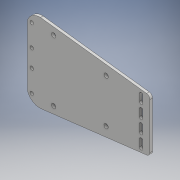
# Autodesk Inventor part: SoporteMano
Saved by Autodesk Inventor 2018 (Build 220112000, 112)
## iProperties
Created: 2017-10-02
Part Number: SoporteMano
Material: Genérico
Document SubType Name: Modeling
Designer: Pablo
Density: 1 g/cm^3
Appearance: Valor por defecto
Author: Pablo
Autodesk Inventor part; units mm, degrees
ref_plane "YZ Plane" through (0, 0, 0) normal (1, 0, 0) x (0, 1, 0)
ref_plane "XZ Plane" through (0, 0, 0) normal (0, 1, 0) x (-1, 0, 0)
ref_plane "XY Plane" through (0, 0, 0) normal (0, 0, 1) x (1, 0, 0)
sketch "Boceto1" plane through (0, 0, 0) normal (0, 1, 0) x (-1, 0, 0)
  line L0 (125, 0) -> (125, 45)
  line L1 (140, 0) -> (140, 35)
  arc A0 (140, 35) -> (125, 45) centre (125.919, 30.1285) ccw
  line L2 (0, 0) -> (0, 26.2041)
  line L3 (10, 0) -> (10, 32.2222)
  line L4 (0, 0) -> (0, 7.5)
  line L5 (0, 7.5) -> (0, 22.5)
  arc A1 (8, 3.5) -> (12, 3.5) centre (10, 3.5) ccw
  line L6 (10, 7.5) -> (6.5727, 7.5)
  arc A2 (12, 11.5) -> (8, 11.5) centre (10, 11.5) ccw
  line L7 (10, 15) -> (5.5099, 15)
  line L8 (12, 11.5) -> (12, 3.5)
  line L9 (8, 3.5) -> (8, 11.5)
  arc A3 (12, 26.5) -> (8, 26.5) centre (10, 26.5) ccw
  arc A4 (8, 18.5) -> (12, 18.5) centre (10, 18.5) ccw
  line L10 (12, 18.5) -> (12, 26.5)
  line L11 (8, 26.5) -> (8, 18.5)
  circle A5 centre (135, 10) radius 2
  circle A6 centre (135, 35) radius 2
  circle A7 centre (110, 35) radius 2.5
  line L12 (125, 45) -> (3.7689, 30.4523)
  circle A8 centre (50, 25) radius 2.5
  arc A9 (3.7689, 30.4523) -> (0, 26.2041) centre (4.2786, 26.2041) ccw
  line L13 (0, 0) -> (10, 0)
  line L14 (125, 0) -> (125, -45)
  line L15 (140, 0) -> (140, -35)
  arc A10 (125, -45) -> (140, -35) centre (125.919, -30.1285) ccw
  line L16 (0, 0) -> (0, -26.2041)
  line L17 (10, 0) -> (10, -32.2222)
  line L18 (0, 0) -> (0, -7.5)
  line L19 (0, -7.5) -> (0, -22.5)
  arc A11 (12, -3.5) -> (8, -3.5) centre (10, -3.5) ccw
  line L20 (10, -7.5) -> (6.5727, -7.5)
  arc A12 (8, -11.5) -> (12, -11.5) centre (10, -11.5) ccw
  line L21 (10, -15) -> (5.5099, -15)
  line L22 (12, -11.5) -> (12, -3.5)
  line L23 (8, -3.5) -> (8, -11.5)
  arc A13 (12, -18.5) -> (8, -18.5) centre (10, -18.5) ccw
  line L24 (12, -18.5) -> (12, -26.5)
  line L25 (8, -26.5) -> (8, -18.5)
  arc A14 (8, -26.5) -> (12, -26.5) centre (10, -26.5) ccw
  circle A15 centre (135, -10) radius 2
  circle A16 centre (135, -35) radius 2
  circle A17 centre (110, -35) radius 2.5
  line L26 (125, -45) -> (3.7689, -30.4523)
  circle A18 centre (50, -25) radius 2.5
  arc A19 (0, -26.2041) -> (3.7689, -30.4523) centre (4.2786, -26.2041) ccw
  dimension "d15" = 45
  dimension "d18" = 15
  dimension "d19" = 35
  dimension "d24" = 140
  dimension "d27" = 10
  dimension "d28" = 7.5
  dimension "d29" = 15
  dimension "d32" = 4
  dimension "d33" = 4
  dimension "d34" = 5
  dimension "d35" = 5
  dimension "d36" = 35
  dimension "d37" = 10
  dimension "d38" = 4
  dimension "d39" = 4
  dimension "d40" = 35
  dimension "d41" = 30
  dimension "d42" = 5
  dimension "d43" = 25
  dimension "d44" = 50
  dimension "d45" = 96.843
  dimension "d51" = 5
  constraints: 54 end point, 36 symmetric about line, 24 point on circle, 20 centre point, 8 point on line, 5 vertical, 3 horizontal, 1 parallel, 1 tangent, 13 other
  measures "d15" distance of L0.start L0.end
  measures "d18" distance between parallel lines of L0 L1
  measures "d19" distance of L1.start L1.end
  measures "d24" distance from line of L1 L2.start
  measures "d27" distance between parallel lines of L3 L2
  measures "d28" distance of L2.start L4.end
  measures "d29" distance of L4.end L5.end
  measures "d32" diameter of A1
  measures "d33" distance from line of L6 A1.centre
  measures "d34" distance from line of L1 A5.centre
  measures "d35" distance from line of L1 A6.centre
  measures "d36" vertical distance of L1.start A6.centre
  measures "d37" vertical distance of L1.start A5.centre
  measures "d38" diameter of A5
  measures "d39" diameter of A6
  measures "d40" vertical distance of L1.start A7.centre
  measures "d41" distance from line of L1 A7.centre
  measures "d42" diameter of A7
  measures "d43" vertical distance of L2.start A8.centre
  measures "d44" distance from line of L2 A8.centre
  measures "d45" angle of L2 L12
  measures "d51" diameter of A8
extrude "Extrusión1" add sketch "Boceto1" along normal blind 3 contours L14 L26 L17 A14 L24 A13 A12 L22 A11 L3 A1 L8 A2 A4 L10 A3 L12 L0 | L0 A0 L1 L15 A10 L14 | L3 A3 L11 A4 A2 L9 A1 L13 L2 A9 L12 | L26 A19 L16 L13 L17 A11 L23 A12 A13 L25 A14
equation "\"d35\" = d34"
